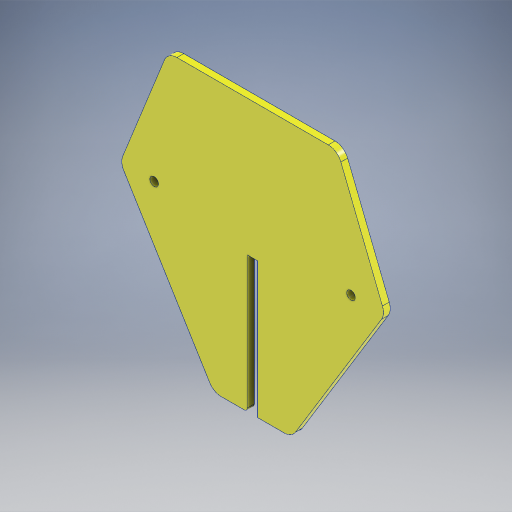
# Autodesk Inventor part: link7
Saved by Autodesk Inventor 2024.1 (Build 281209000, 209)
## iProperties
Created: 2023-09-09
Part Number: link7
Material: Aluminum 6061
Document SubType Name: Modeling
Designer: Camilo
Density: 2.7 g/cm^3
Appearance: Aluminum - Flat
Mass: 23.6363 g
Surface Area: 94.4708 cm^2
Volume: 8.75417 cm^3
Author: Camilo
Autodesk Inventor part; units mm, degrees
ref_plane "YZ Plane" through (0, 0, 0) normal (1, 0, 0) x (0, 1, 0)
ref_plane "XZ Plane" through (0, 0, 0) normal (0, 1, 0) x (-1, 0, 0)
ref_plane "XY Plane" through (0, 0, 0) normal (0, 0, 1) x (1, 0, 0)
sketch "Sketch6" plane through (0, 0, 0) normal (0, 0, 1) x (1, 0, 0)
  line L0 (0, 0) -> (0, 20)
  line L1 (0, 0) -> (0, -19)
  line L2 (0, 20) -> (29, 20)
  line L3 (29, 20) -> (29, 25)
  line L4 (0, 20) -> (-29, 20)
  line L5 (-29, 20) -> (-29, 25)
  circle A0 centre (-29, 25) radius 1.25
  circle A1 centre (29, 25) radius 1.25
  line L6 (-29, 25) -> (-39, 25)
  line L7 (29, 25) -> (39, 25)
  line L8 (0, 20) -> (1.5, 20)
  line L9 (1.5, 20) -> (-1.5, 20)
  line L10 (-1.5, 20) -> (-1.5, -19)
  line L11 (1, -20) -> (1.5, -20)
  line L12 (1.5, -20) -> (1.5, 20)
  line L13 (1.5, -20) -> (9.2567, -20)
  line L14 (-2.5, -20) -> (-9.2567, -20)
  line L15 (-37.9548, 23.2897) -> (-12.6698, -18.0858)
  line L16 (37.9548, 23.2897) -> (12.6698, -18.0858)
  arc A2 (-12.6698, -18.0858) -> (-9.2567, -20) centre (-9.2567, -16) ccw
  arc A3 (9.2567, -20) -> (12.6698, -18.0858) centre (9.2567, -16) ccw
  arc A4 (0, -19) -> (1, -20) centre (1, -19) ccw
  arc A5 (-2.5, -20) -> (-1.5, -19) centre (-2.5, -19) ccw
  line L17 (0, 20) -> (0, 60)
  line L18 (0, 60) -> (22.2919, 60)
  line L19 (0, 60) -> (-22.2919, 60)
  line L20 (-26.0058, 57.4856) -> (-38.2556, 26.861)
  line L21 (26.0058, 57.4856) -> (38.2556, 26.861)
  arc A6 (-38.2556, 26.861) -> (-37.9548, 23.2897) centre (-34.5417, 25.3755) ccw
  arc A7 (37.9548, 23.2897) -> (38.2556, 26.861) centre (34.5417, 25.3755) ccw
  arc A8 (26.0058, 57.4856) -> (22.2919, 60) centre (22.2919, 56) ccw
  arc A9 (-22.2919, 60) -> (-26.0058, 57.4856) centre (-22.2919, 56) ccw
  point P0 (0, -20)
  point P1 (-1.5, -20)
  point P2 (11.5, -20)
  point P3 (-11.5, -20)
  point P4 (25, 60)
  point P5 (-25, 60)
  dimension "d115" = 20
  dimension "d116" = 20
  dimension "d117" = 29
  dimension "d118" = 5
  dimension "d119" = 5
  dimension "d120" = 29
  dimension "d121" = 2.5
  dimension "d122" = 2.5
  dimension "d123" = 10
  dimension "d124" = 10
  dimension "d125" = 1.5
  dimension "d126" = 3
  dimension "d127" = 10
  dimension "d128" = 10
  dimension "d129" = 4
  dimension "d130" = 1
  dimension "d131" = 40
  dimension "d132" = 25
  dimension "d133" = 25
  dimension "d134" = 4
  constraints: 44 end point, 17 point on line, 16 point on circle, 16 tangent, 10 centre point, 8 horizontal, 5 equal radius, 4 perpendicular, 3 vertical, 2 coincident, 2 parallel
  measures "d115" distance of L0.start L0.end
  measures "d116" distance of L0.start point (0, -20)
  measures "d117" distance of L0.end L2.end
  measures "d118" distance of L2.end L3.end
  measures "d119" distance of L4.end L5.end
  measures "d120" distance of L0.end L4.end
  measures "d121" diameter of A0
  measures "d122" diameter of A1
  measures "d123" distance of L6.start L6.end
  measures "d124" distance of L7.start L7.end
  measures "d125" distance of L0.end L8.end
  measures "d126" distance of L11.end point (-1.5, -20)
  measures "d127" distance of L11.end point (11.5, -20)
  measures "d128" distance of point (-1.5, -20) point (-11.5, -20)
  measures "d129" radius of A2
  measures "d130" radius of A4
  measures "d131" distance of L0.end L17.end
  measures "d132" distance of L17.end point (25, 60)
  measures "d133" distance of L17.end point (-25, 60)
  measures "d134" radius of A6
extrude "Extrusion8" add sketch "Sketch6" along normal mid plane 2 contours L17 L18 A8 L21 A7 L7 A1 L3 L2 | L4 L5 A0 L6 A6 L20 A9 L19 L17 | L2 L3 A1 L7 A7 L16 A3 L13 L12 | L10 A5 L14 A2 L15 A6 L6 A0 L5 L4
body "Solid3"
